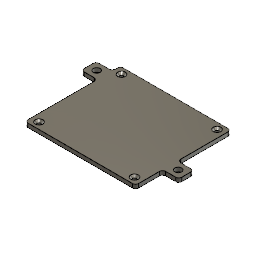
Power PCB Bracket v2 (Autodesk Fusion 360 design; units mm, degrees)
Autodesk Fusion 360 part; units mm, degrees
sketch "Sketch1" plane through (0, 0, 0) normal (0, 1, 0) x (1, 0, 0)
  line L0 (47.35, 40.9) -> (-47.35, 40.9) construction
  line L1 (-47.35, 40.9) -> (-47.35, -40.9) construction
  line L2 (-47.35, -40.9) -> (47.35, -40.9) construction
  line L3 (47.35, -40.9) -> (47.35, 40.9) construction
  line L4 (47.35, 40.9) -> (-47.35, -40.9) construction
  line L5 (-47.35, 40.9) -> (47.35, -40.9) construction
  line L6 (54.9177, 47.4368) -> (-54.9177, 47.4368)
  line L7 (-54.9177, 47.4368) -> (-54.9177, -47.4368)
  line L8 (-54.9177, -47.4368) -> (54.9177, -47.4368)
  line L9 (54.9177, -47.4368) -> (54.9177, 47.4368)
  line L10 (54.9177, 47.4368) -> (-54.9177, -47.4368) construction
  line L11 (-54.9177, 47.4368) -> (54.9177, -47.4368) construction
  circle A0 centre (47.35, 40.9) radius 1.75
  line L12 (0, 0) -> (0, 35) construction
  line L13 (0, 0) -> (-41.0628, 0) construction
  circle A1 centre (-47.35, 40.9) radius 1.75
  circle A2 centre (47.35, -40.9) radius 1.75
  circle A3 centre (-47.35, -40.9) radius 1.75
  line L14 (-54.9177, 39.4) -> (-70.9177, 39.4)
  line L15 (-70.9177, 39.4) -> (-70.9177, 24.4)
  line L16 (-70.9177, 24.4) -> (-54.9177, 24.4)
  line L17 (-54.9177, 24.4) -> (-54.9177, 39.4)
  line L18 (54.9177, -5.6) -> (70.9177, -5.6)
  line L19 (70.9177, -5.6) -> (70.9177, -20.6)
  line L20 (70.9177, -20.6) -> (54.9177, -20.6)
  line L21 (54.9177, -20.6) -> (54.9177, -5.6)
  line L22 (81.8257, 31.9) -> (62.2169, 31.9) construction
  line L23 (80.3912, -13.1) -> (59.348, -13.1) construction
  circle A4 centre (-62.9177, 31.9) radius 3.4
  circle A5 centre (62.9177, -13.1) radius 3.4
  dimension "d1" = 3.5
  dimension "d2" = 81.8
  dimension "d3" = 94.7
  dimension "d4" = 10
  dimension "d5" = 16
  dimension "d6" = 15
  dimension "d7" = 15
  dimension "d9" = 16
  dimension "d10" = 45
  dimension "d11" = 9
  dimension "d12" = 6.8
  dimension "d13" = 6.8
  dimension "d14" = 8
  dimension "d15" = 8
  constraint perpendicular L0 L1
  constraint parallel L0 L2
  constraint parallel L1 L3
  constraint horizontal L0
  constraint coincident L4 L12.start
  constraint coincident L5 L12.start
  constraint coincident L12.start L13.start
  constraint perpendicular L6 L7
  constraint parallel L6 L8
  constraint parallel L7 L9
  constraint horizontal L6
  constraint coincident L10 L12.start
  constraint coincident L11 L12.start
  constraint collinear L4 L10
  constraint coincident L0.start L3.end
  constraint vertical L12
  constraint horizontal L13
  constraint symmetric A0 L12 A1
  constraint symmetric A0 L13 A2
  constraint symmetric L13 A1 A3
  constraint horizontal L14
  constraint vertical L15
  constraint horizontal L16
  constraint vertical L17
  constraint coincident L7 L14.start
  constraint horizontal L18
  constraint vertical L19
  constraint horizontal L20
  constraint vertical L21
  constraint coincident L9 L18.start
  constraint perpendicular L12 L22
  constraint symmetric L14 L16 L22
  constraint symmetric L18 L20 L23
  constraint coincident L23 A5.centre
  constraint coincident L22 A4.centre
  measures "d1" diameter of A0
  measures "d2" distance of L0.start L2.end
  measures "d3" distance of L0.start L0.end
  measures "d4" distance of L6.start L0.start
  measures "d5" distance of L14.start L14.end
  measures "d6" distance of L14.end L15.end
  measures "d7" distance of L18.end L19.end
  measures "d9" distance of L18.start L18.end
  measures "d10" distance of L22 L23
  measures "d11" distance of L0.end L22
  measures "d12" diameter of A5
  measures "d13" diameter of A4
  measures "d14" distance of L7 A4.centre
  measures "d15" distance of L21 A5.centre
extrude "Extrude1" add sketch "Sketch1" along normal blind 4
fillet "Fillet1" radius 3 12 edges at (-70.9177, 2, -24.4) (-70.9177, 2, -39.4) (-54.9177, 2, -39.4) (-54.9177, 2, -47.4368) (-54.9177, 2, 47.4368) (-54.9177, 2, -24.4) (54.9177, 2, 47.4368) (54.9177, 2, 20.6) (70.9177, 2, 20.6) (70.9177, 2, 5.6) (54.9177, 2, 5.6) (54.9177, 2, -47.4368)
chamfer "Chamfer1" distance 2 angle 45 4 edges at (45.7184, 4, 40.2672) (-48.9816, 4, 40.2672) (-48.9816, 4, -41.5328) (45.7184, 4, -41.5328)
